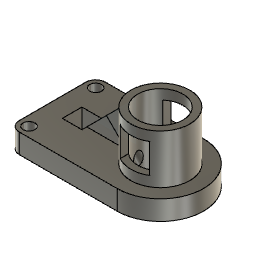
drawing_2 v2 (Autodesk Fusion 360 design; units mm, degrees)
Autodesk Fusion 360 part; units mm, degrees
note: some values were not read from the file. Set by a fixed rule: which sketch regions a step uses.
sketch "Sketch1" plane through (0, 0, 0) normal (0, 0, 1) x (1, 0, 0)
  line L0 (0, 0) -> (-100, 0)
  line L1 (-100, 0) -> (-100, 10)
  line L2 (-100, 10) -> (-110, 10)
  circle A0 centre (-100, 10) radius 10
  circle A1 centre (-100, 10) radius 6
  line L3 (-110, 10) -> (-110, 78)
  line L4 (-110, 78) -> (-100, 78)
  line L5 (-100, 78) -> (-100, 88)
  circle A2 centre (-100, 78) radius 10
  circle A3 centre (-100, 78) radius 6
  line L6 (-100, 88) -> (0, 88)
  line L7 (0, 88) -> (0, 0)
  circle A4 centre (0, 44) radius 44
  line L8 (0, 44) -> (-110, 44)
  line L9 (-110, 44) -> (-80, 44)
  line L10 (-80, 44) -> (-70, 44)
  line L11 (-70, 44) -> (-70, 34)
  line L12 (-70, 34) -> (-80, 34)
  line L13 (-80, 34) -> (-80, 44)
  line L14 (-80, 44) -> (-70, 44)
  line L15 (-70, 44) -> (-70, 54)
  line L16 (-70, 54) -> (-80, 54)
  line L17 (-80, 54) -> (-80, 44)
  line L18 (-80, 44) -> (-90, 44)
  line L19 (-90, 44) -> (-90, 54)
  line L20 (-90, 54) -> (-80, 54)
  line L21 (-80, 54) -> (-80, 44)
  line L22 (-80, 44) -> (-90, 44)
  line L23 (-90, 44) -> (-90, 34)
  line L24 (-90, 34) -> (-80, 34)
  line L25 (-80, 34) -> (-80, 44)
  dimension "d1" = 100
  dimension "d2" = 10
  dimension "d3" = 10
  dimension "d4" = 20
  dimension "d5" = 12
  dimension "d6" = 68
  dimension "d7" = 10
  dimension "d8" = 10
  dimension "d9" = 20
  dimension "d10" = 12
  dimension "d11" = 100
  dimension "d12" = 88
  dimension "d13" = 30
  dimension "d14" = 10
  dimension "d15" = 10
  dimension "d16" = 10
  dimension "d17" = 10
  dimension "d18" = 10
  dimension "d19" = 10
  dimension "d20" = 10
  dimension "d21" = 10
  constraint coincident L0.start L7.end
  constraint horizontal L0
  constraint perpendicular L0 L1
  constraint perpendicular L1 L2
  constraint coincident L1.end L2.start
  constraint concentric A0 A1
  constraint perpendicular L2 L3
  constraint perpendicular L3 L4
  constraint perpendicular L4 L5
  constraint coincident L4.end L5.start
  constraint concentric A2 A3
  constraint perpendicular L5 L6
  constraint midpoint L7 A4.centre
  constraint coincident A4.centre L8.start
  constraint midpoint L3 L8.end
  constraint perpendicular L3 L9
  constraint horizontal L10
  constraint vertical L11
  constraint horizontal L12
  constraint vertical L13
  constraint horizontal L14
  constraint vertical L15
  constraint horizontal L16
  constraint vertical L17
  constraint horizontal L18
  constraint vertical L19
  constraint horizontal L20
  constraint vertical L21
  constraint horizontal L22
  constraint vertical L23
  constraint horizontal L24
  constraint vertical L25
  measures "d1" distance of L0.start L0.end
  measures "d2" distance of L0.end L1.end
  measures "d3" distance of L1.end L2.end
  measures "d4" diameter of A0
  measures "d5" diameter of A1
  measures "d6" distance of L2.end L3.end
  measures "d7" distance of L3.end L4.end
  measures "d8" distance of L4.end L5.end
  measures "d9" diameter of A2
  measures "d10" diameter of A3
  measures "d11" distance of L5.end L6.end
  measures "d12" diameter of A4
  measures "d13" distance of L8.end L9.end
  measures "d14" distance of L9.end L10.end
  measures "d15" distance of L9.end L12.end
  measures "d16" distance of L9.end L10.end
  measures "d17" distance of L9.end L16.end
  measures "d18" distance of L9.end L18.end
  measures "d19" distance of L9.end L16.end
  measures "d20" distance of L9.end L18.end
  measures "d21" distance of L9.end L12.end
extrude "Extrude1" add sketch "Sketch1" along normal blind 20 contours L7 A4 L8 | L7 A4 | L0 A0 L3 A4 L8 L9 L11 L12 L23 L24 | L1 L2 A0 A1 | L1 L2 A0 A1 | L7 A4 L8 | L3 A2 L6 A4 L8 L9 L15 L16 L19 L20 | L4 L5 A2 A3 | L4 L5 A2 A3 makes body 1
sketch "Sketch2" plane through (0, 0, 20) normal (0, 0, 1) x (-1, 0, 0)
  circle A0 centre (100, -10) radius 6
  circle A1 centre (100, -78) radius 6
  line L0 (90, -34) -> (90, -54)
  line L1 (90, -54) -> (70, -54)
  line L2 (70, -54) -> (70, -34)
  line L3 (70, -34) -> (90, -34)
  arc A2 (110, -10) -> (100, 0) centre (100, -10) ccw
  line L4 (100, 0) -> (0, 0)
  arc A3 (0, 0) -> (0, -88) centre (0, -44) ccw
  line L5 (0, -88) -> (100, -88)
  arc A4 (100, -88) -> (110, -78) centre (100, -78) ccw
  line L6 (110, -78) -> (110, -10)
  line L7 (0, 0) -> (0, -88)
  line L8 (110, -44) -> (0, -44)
  circle A5 centre (0, -44) radius 30
  circle A6 centre (0, -44) radius 23
  dimension "d24" = 60
  dimension "d25" = 46
  constraint coincident L4.end A3.start
  constraint coincident A3.end L5.start
  constraint midpoint L6 L8.start
  constraint coincident A3.centre L8.end
  measures "d24" diameter of A5
  measures "d25" diameter of A6
extrude "Extrude2" add sketch "Sketch2" along normal blind 50 contours L7 L8 A5 A6 | L7 L8 A5 A6 | L7 A5 A6 bodies 1
extrude "Extrude3" cut 1 faces at (5.9607, 51.4744, 20) along direction (0, 0, -1) blind 20 on bodies 1 bodies 1
sketch "Sketch3" plane through (0, 0, 0) normal (0, 1, 0) x (1, 0, 0)
  line L0 (0, -60) -> (-15, -60)
  line L1 (-15, -60) -> (-15, -30)
  line L2 (-15, -30) -> (0, -30)
  line L3 (0, -30) -> (0, -60)
  line L4 (0, -60) -> (15, -60)
  line L5 (15, -60) -> (15, -30)
  line L6 (15, -30) -> (0, -30)
  line L7 (0, -30) -> (0, -60)
  dimension "d31" = 15
  dimension "d32" = 30
  dimension "d33" = 30
  constraint horizontal L0
  constraint vertical L1
  constraint horizontal L2
  constraint vertical L3
  constraint horizontal L4
  constraint vertical L5
  constraint horizontal L6
  constraint vertical L7
  measures "d31" distance of L0.start L0.end
  measures "d32" distance of L0.start L2.end
  measures "d33" distance of L0.start L2.end
extrude "Extrude4" cut sketch "Sketch3" along normal blind 95 bodies 1
sketch "Sketch4" plane through (0, 0, 0) normal (0, 1, 0) x (1, 0, 0)
ref_plane "WorkPlane1" through (-50, 44, 10) normal (0, 1, 0) x (-1, 0, 0)
sketch "Sketch5" plane through (-50, 44, 10) normal (0, 1, 0) x (1, 0, 0)
  line L0 (20, -10) -> (20, -50)
  line L1 (20, -10) -> (-20, -10)
  line L2 (-20, -10) -> (20, -50)
  constraint vertical L0
  constraint perpendicular L0 L1
extrude "Extrude5" add sketch "Sketch5" along normal mid plane 10 separate body makes body 2
sketch "Sketch6" plane through (0, 49, 0) normal (0, 1, 0) x (-1, 0, 0)
  line L0 (30, 20) -> (70, 20)
  line L1 (70, 20) -> (30, 60)
  line L2 (30, 60) -> (30, 20)
sketch "Sketch7" plane through (-45, 0, 45) normal (-0.707107, 0, 0.707107) x (0, -1, 0)
  line L0 (-39, 21.2132) -> (-49, 21.2132)
  line L1 (-49, 21.2132) -> (-49, -35.3553)
  line L2 (-49, -35.3553) -> (-39, -35.3553)
  line L3 (-39, -35.3553) -> (-39, 21.2132)
  line L4 (-49, -7.0711) -> (-39, -7.0711)
  circle A0 centre (-44, -7.0711) radius 5
  dimension "d39" = 10
  constraint midpoint L1 L4.start
  constraint midpoint L3 L4.end
  constraint midpoint L4 A0.centre
  measures "d39" diameter of A0
extrude "Extrude6" cut sketch "Sketch7" against normal blind 145 contours L4 A0 | L4 A0 bodies 1 2
